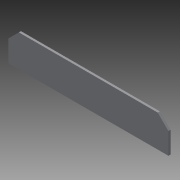
# Autodesk Inventor part: autorzy projektu
Saved by Autodesk Inventor 2014 (Build 180170000, 170)
## iProperties
Created: 2018-03-11
Part Number: autorzy projektu
Material: Generic
Document SubType Name: Modeling
Designer: HP820
Density: 1 g/cm^3
Appearance: Default
Author: HP820
Autodesk Inventor part; units mm, degrees
ref_plane "YZ Plane" through (0, 0, 0) normal (1, 0, 0) x (0, 1, 0)
ref_plane "XZ Plane" through (0, 0, 0) normal (0, 1, 0) x (-1, 0, 0)
ref_plane "XY Plane" through (0, 0, 0) normal (0, 0, 1) x (1, 0, 0)
sketch "Sketch1" plane through (0, 0, 0) normal (0, 1, 0) x (-1, 0, 0)
  line L0 (-75, 15) -> (75, 15)
  line L1 (75, 15) -> (75, -15)
  line L2 (75, -15) -> (-75, -15)
  line L3 (-75, -15) -> (-75, 15)
  line L4 (-75, 15) -> (75, -15) construction
  line L5 (75, 15) -> (-75, -15) construction
  point P0 (0, 0)
  dimension "d0" = 150
  dimension "d1" = 30
  constraints: 12 end point, 2 midpoint, 2 parallel, 1 horizontal, 1 perpendicular
  measures "d0" distance of L1.end L2.end
  measures "d1" distance of L0.end L1.end
extrude "Extrusion1" add sketch "Sketch1" along normal blind 2
chamfer "Chamfer1" distance 10 angle 45 2 edges at (75, 1, 15) (-75, 1, 15)
sketch "Sketch2" plane through (0, 2, 0) normal (0, 1, 0) x (1, 0, 0)
  line L0 (74.6856, -7.7413) -> (-73.3171, -7.7413) construction
  line L1 (-73.3171, -7.7413) -> (-73.3171, 7.0993) construction
  line L2 (-73.3171, 7.0993) -> (74.6856, 7.0993) construction
  line L3 (74.6856, 7.0993) -> (74.6856, -7.7413) construction
  spline S0 degree 2 poles (34.3952, -8.515) (34.3952, -8.0272) (35.3438, -8.0272) knots 0 0 0 1 1 1
  line L4 (35.3438, -8.0272) -> (37.8644, -8.0272)
  line L5 (37.8644, -8.0272) -> (37.8644, -6.1454)
  line L6 (37.8644, -6.1454) -> (39.4209, -6.1454)
  line L7 (39.4209, -6.1454) -> (39.4209, -11.3454)
  line L8 (39.4209, -11.3454) -> (35.3438, -11.3454)
  spline S1 degree 2 poles (35.3438, -11.3454) (34.3952, -11.3454) (34.3952, -10.8653) knots 0 0 0 1 1 1
  line L9 (34.3952, -10.8653) -> (34.3952, -8.515)
  line L10 (35.9633, -8.697) -> (35.9633, -10.6756)
  line L11 (35.9633, -10.6756) -> (37.8644, -10.6756)
  line L12 (37.8644, -10.6756) -> (37.8644, -8.697)
  line L13 (37.8644, -8.697) -> (35.9633, -8.697)
  line L14 (29.1371, -8.0969) -> (30.6433, -8.0969)
  line L15 (30.6433, -8.0969) -> (30.6433, -8.8674)
  line L16 (30.6433, -8.8674) -> (31.8474, -8.8519)
  line L17 (31.8474, -8.8519) -> (31.8474, -6.1454)
  line L18 (31.8474, -6.1454) -> (33.3691, -6.1454)
  line L19 (33.3691, -6.1454) -> (33.3691, -9.4985)
  line L20 (33.3691, -9.4985) -> (31.8474, -9.4985)
  line L21 (31.8474, -9.4985) -> (31.8474, -9.3785)
  spline S2 degree 2 poles (31.8474, -9.3785) (31.3751, -9.4211) (30.9104, -9.4637) knots 0 0 0 1 1 1
  spline S3 degree 2 poles (30.9104, -9.4637) (30.3451, -9.514) (29.9657, -9.514) knots 0 0 0 1 1 1
  spline S4 degree 2 poles (29.9657, -9.514) (29.1371, -9.514) (29.1371, -9.1036) knots 0 0 0 1 1 1
  line L22 (29.1371, -9.1036) -> (29.1371, -8.0969)
  spline S5 degree 2 poles (23.8519, -6.5597) (23.8519, -6.1454) (24.696, -6.1454) knots 0 0 0 1 1 1
  line L23 (24.696, -6.1454) -> (27.4218, -6.1454)
  spline S6 degree 2 poles (27.4218, -6.1454) (28.2775, -6.1454) (28.2775, -6.5597) knots 0 0 0 1 1 1
  line L24 (28.2775, -6.5597) -> (28.2775, -9.0842)
  spline S7 degree 2 poles (28.2775, -9.0842) (28.2775, -9.4985) (27.4218, -9.4985) knots 0 0 0 1 1 1
  line L25 (27.4218, -9.4985) -> (24.696, -9.4985)
  spline S8 degree 2 poles (24.696, -9.4985) (23.8519, -9.4985) (23.8519, -9.0842) knots 0 0 0 1 1 1
  line L26 (23.8519, -9.0842) -> (23.8519, -6.5597)
  line L27 (25.3387, -6.7765) -> (25.3387, -8.8674)
  line L28 (25.3387, -8.8674) -> (26.783, -8.8674)
  line L29 (26.783, -8.8674) -> (26.783, -6.7765)
  line L30 (26.783, -6.7765) -> (25.3387, -6.7765)
  spline S9 degree 2 poles (21.219, -5.3362) (21.219, -4.918) (22.0631, -4.918) knots 0 0 0 1 1 1
  line L31 (22.0631, -4.918) -> (23.6777, -4.918)
  line L32 (23.6777, -4.918) -> (23.6777, -5.553)
  line L33 (23.6777, -5.553) -> (22.7136, -5.553)
  line L34 (22.7136, -5.553) -> (22.7136, -9.4985)
  line L35 (22.7136, -9.4985) -> (21.219, -9.4985)
  line L36 (21.219, -9.4985) -> (21.219, -5.3362)
  line L37 (21.2035, -9.9825) -> (22.7252, -9.9825)
  line L38 (22.7252, -9.9825) -> (22.7252, -10.7646)
  line L39 (22.7252, -10.7646) -> (21.2035, -10.7646)
  line L40 (21.2035, -10.7646) -> (21.2035, -9.9825)
  spline S10 degree 2 poles (15.7441, -6.5597) (15.7441, -6.1454) (16.6037, -6.1454) knots 0 0 0 1 1 1
  line L41 (16.6037, -6.1454) -> (19.2288, -6.1454)
  spline S11 degree 2 poles (19.2288, -6.1454) (20.0845, -6.1454) (20.0845, -6.5597) knots 0 0 0 1 1 1
  line L42 (20.0845, -6.5597) -> (20.0845, -9.0842)
  spline S12 degree 2 poles (20.0845, -9.0842) (20.0845, -9.4985) (19.2288, -9.4985) knots 0 0 0 1 1 1
  line L43 (19.2288, -9.4985) -> (16.6037, -9.4985)
  spline S13 degree 2 poles (16.6037, -9.4985) (15.7441, -9.4985) (15.7441, -9.0842) knots 0 0 0 1 1 1
  line L44 (15.7441, -9.0842) -> (15.7441, -7.8529)
  line L45 (15.7441, -7.8529) -> (16.1623, -7.6438)
  line L46 (16.1623, -7.6438) -> (18.6287, -7.6438)
  line L47 (18.6287, -7.6438) -> (18.6287, -6.703)
  line L48 (18.6287, -6.703) -> (17.1999, -6.703)
  line L49 (17.1999, -6.703) -> (17.1999, -7.2605)
  line L50 (17.1999, -7.2605) -> (15.7441, -7.2605)
  line L51 (15.7441, -7.2605) -> (15.7441, -6.5597)
  line L52 (17.1999, -8.1395) -> (17.1999, -8.9409)
  line L53 (17.1999, -8.9409) -> (18.6287, -8.9409)
  line L54 (18.6287, -8.9409) -> (18.6287, -8.1395)
  line L55 (18.6287, -8.1395) -> (17.1999, -8.1395)
  line L56 (10.1608, -6.1454) -> (11.7831, -6.1454)
  line L57 (11.7831, -6.1454) -> (13.1189, -7.6826)
  line L58 (13.1189, -7.6826) -> (13.1189, -6.1454)
  line L59 (13.1189, -6.1454) -> (14.6406, -6.1454)
  line L60 (14.6406, -6.1454) -> (14.6406, -11.3454)
  line L61 (14.6406, -11.3454) -> (13.1189, -11.3454)
  line L62 (13.1189, -11.3454) -> (13.1189, -8.2208)
  line L63 (13.1189, -8.2208) -> (11.9148, -9.4985)
  line L64 (11.9148, -9.4985) -> (10.3273, -9.4985)
  line L65 (10.3273, -9.4985) -> (10.3273, -9.4869)
  line L66 (10.3273, -9.4869) -> (11.876, -7.9613)
  line L67 (11.876, -7.9613) -> (10.1608, -6.1454)
  line L68 (6.6102, -6.1454) -> (8.2984, -6.1454)
  spline S14 degree 2 poles (8.2984, -6.1454) (9.1425, -6.1454) (9.1425, -6.5597) knots 0 0 0 1 1 1
  line L69 (9.1425, -6.5597) -> (9.1425, -8.8519)
  line L70 (9.1425, -8.8519) -> (9.8588, -8.8519)
  line L71 (9.8588, -8.8519) -> (9.8588, -9.4985)
  line L72 (9.8588, -9.4985) -> (9.1425, -9.4985)
  line L73 (9.1425, -9.4985) -> (9.1425, -10.4123)
  line L74 (9.1425, -10.4123) -> (7.6247, -10.4123)
  line L75 (7.6247, -10.4123) -> (7.6247, -9.4985)
  line L76 (7.6247, -9.4985) -> (6.6489, -9.4985)
  line L77 (6.6489, -9.4985) -> (6.6489, -8.8519)
  line L78 (6.6489, -8.8519) -> (7.6247, -8.8519)
  line L79 (7.6247, -8.8519) -> (7.6247, -6.792)
  line L80 (7.6247, -6.792) -> (6.6102, -6.792)
  line L81 (6.6102, -6.792) -> (6.6102, -6.1454)
  line L82 (-3.6852, -9.4985) -> (-2.241, -6.1377)
  line L83 (-2.241, -6.1377) -> (-0.9129, -6.1377)
  line L84 (-0.9129, -6.1377) -> (-0.1889, -7.9962)
  line L85 (-0.1889, -7.9962) -> (0.5352, -6.1377)
  line L86 (0.5352, -6.1377) -> (1.8516, -6.1377)
  line L87 (1.8516, -6.1377) -> (3.2958, -9.4985)
  line L88 (3.2958, -9.4985) -> (1.84, -9.4985)
  line L89 (1.84, -9.4985) -> (1.1082, -7.3573)
  line L90 (1.1082, -7.3573) -> (0.3842, -9.4985)
  line L91 (0.3842, -9.4985) -> (-0.7736, -9.4985)
  line L92 (-0.7736, -9.4985) -> (-1.4976, -7.3573)
  line L93 (-1.4976, -7.3573) -> (-2.2294, -9.4985)
  line L94 (-2.2294, -9.4985) -> (-3.6852, -9.4985)
  line L95 (-8.982, -9.4985) -> (-7.3016, -6.188)
  line L96 (-7.3016, -6.188) -> (-6.655, -4.918)
  line L97 (-6.655, -4.918) -> (-5.0985, -4.918)
  line L98 (-5.0985, -4.918) -> (-5.7993, -6.1725)
  line L99 (-5.7993, -6.1725) -> (-4.0957, -9.4985)
  line L100 (-4.0957, -9.4985) -> (-5.6599, -9.4985)
  line L101 (-5.6599, -9.4985) -> (-6.5427, -7.2954)
  line L102 (-6.5427, -7.2954) -> (-7.4255, -9.4985)
  line L103 (-7.4255, -9.4985) -> (-8.982, -9.4985)
  line L104 (-14.213, -6.1454) -> (-12.5907, -6.1454)
  line L105 (-12.5907, -6.1454) -> (-11.2549, -7.6826)
  line L106 (-11.2549, -7.6826) -> (-11.2549, -6.1454)
  line L107 (-11.2549, -6.1454) -> (-9.7332, -6.1454)
  line L108 (-9.7332, -6.1454) -> (-9.7332, -11.3454)
  line L109 (-9.7332, -11.3454) -> (-11.2549, -11.3454)
  line L110 (-11.2549, -11.3454) -> (-11.2549, -8.2208)
  line L111 (-11.2549, -8.2208) -> (-12.459, -9.4985)
  line L112 (-12.459, -9.4985) -> (-14.0465, -9.4985)
  line L113 (-14.0465, -9.4985) -> (-14.0465, -9.4869)
  line L114 (-14.0465, -9.4869) -> (-12.4978, -7.9613)
  line L115 (-12.4978, -7.9613) -> (-14.213, -6.1454)
  spline S15 degree 2 poles (-19.293, -6.5597) (-19.293, -6.1454) (-18.4489, -6.1454) knots 0 0 0 1 1 1
  line L116 (-18.4489, -6.1454) -> (-15.7231, -6.1454)
  spline S16 degree 2 poles (-15.7231, -6.1454) (-14.8674, -6.1454) (-14.8674, -6.5597) knots 0 0 0 1 1 1
  line L117 (-14.8674, -6.5597) -> (-14.8674, -9.0842)
  spline S17 degree 2 poles (-14.8674, -9.0842) (-14.8674, -9.4985) (-15.7231, -9.4985) knots 0 0 0 1 1 1
  line L118 (-15.7231, -9.4985) -> (-18.4489, -9.4985)
  spline S18 degree 2 poles (-18.4489, -9.4985) (-19.293, -9.4985) (-19.293, -9.0842) knots 0 0 0 1 1 1
  line L119 (-19.293, -9.0842) -> (-19.293, -6.5597)
  line L120 (-17.8062, -6.7765) -> (-17.8062, -8.8674)
  line L121 (-17.8062, -8.8674) -> (-16.3619, -8.8674)
  line L122 (-16.3619, -8.8674) -> (-16.3619, -6.7765)
  line L123 (-16.3619, -6.7765) -> (-17.8062, -6.7765)
  line L124 (-24.8724, -6.1454) -> (-23.343, -6.1454)
  line L125 (-23.343, -6.1454) -> (-23.343, -8.8674)
  line L126 (-23.343, -8.8674) -> (-21.9143, -8.8519)
  line L127 (-21.9143, -8.8519) -> (-21.9143, -6.1454)
  line L128 (-21.9143, -6.1454) -> (-20.3926, -6.1454)
  line L129 (-20.3926, -6.1454) -> (-20.3926, -9.4985)
  line L130 (-20.3926, -9.4985) -> (-21.9143, -9.4985)
  line L131 (-21.9143, -9.4985) -> (-21.9143, -9.3785)
  spline S19 degree 2 poles (-21.9143, -9.3785) (-22.4447, -9.4211) (-22.9713, -9.4598) knots 0 0 0 1 1 1
  spline S20 degree 2 poles (-22.9713, -9.4598) (-23.6218, -9.514) (-24.04, -9.514) knots 0 0 0 1 1 1
  spline S21 degree 2 poles (-24.04, -9.514) (-24.8724, -9.514) (-24.8724, -9.1036) knots 0 0 0 1 1 1
  line L132 (-24.8724, -9.1036) -> (-24.8724, -6.1454)
  line L133 (-30.2893, -6.1454) -> (-28.8334, -6.1454)
  line L134 (-28.8334, -6.1454) -> (-28.8334, -6.2616)
  spline S22 degree 2 poles (-28.8334, -6.2616) (-28.3185, -6.2228) (-27.7996, -6.1803) knots 0 0 0 1 1 1
  spline S23 degree 2 poles (-27.7996, -6.1803) (-27.122, -6.1338) (-26.7697, -6.1338) knots 0 0 0 1 1 1
  spline S24 degree 2 poles (-26.7697, -6.1338) (-25.9372, -6.1338) (-25.9372, -6.5403) knots 0 0 0 1 1 1
  line L135 (-25.9372, -6.5403) -> (-25.9372, -7.7484)
  spline S25 degree 2 poles (-25.9372, -7.7484) (-25.9372, -8.1666) (-26.7929, -8.1666) knots 0 0 0 1 1 1
  line L136 (-26.7929, -8.1666) -> (-28.8489, -8.1666)
  line L137 (-28.8489, -8.1666) -> (-28.8489, -8.9371)
  line L138 (-28.8489, -8.9371) -> (-27.3931, -8.9371)
  line L139 (-27.3931, -8.9371) -> (-27.3931, -8.457)
  line L140 (-27.3931, -8.457) -> (-26.0185, -8.457)
  line L141 (-26.0185, -8.457) -> (-26.0185, -9.0842)
  spline S26 degree 2 poles (-26.0185, -9.0842) (-26.0185, -9.4985) (-26.8742, -9.4985) knots 0 0 0 1 1 1
  line L142 (-26.8742, -9.4985) -> (-29.4452, -9.4985)
  spline S27 degree 2 poles (-29.4452, -9.4985) (-30.2893, -9.4985) (-30.2893, -9.0842) knots 0 0 0 1 1 1
  line L143 (-30.2893, -9.0842) -> (-30.2893, -6.1454)
  line L144 (-28.8489, -6.7494) -> (-28.8489, -7.6516)
  line L145 (-28.8489, -7.6516) -> (-27.3931, -7.6516)
  line L146 (-27.3931, -7.6516) -> (-27.3931, -6.7223)
  line L147 (-27.3931, -6.7223) -> (-28.8489, -6.7494)
  line L148 (-32.9144, -6.1454) -> (-31.4199, -6.1454)
  line L149 (-31.4199, -6.1454) -> (-31.4199, -11.3454)
  line L150 (-31.4199, -11.3454) -> (-32.9144, -11.3454)
  line L151 (-32.9144, -11.3454) -> (-32.9144, -6.1454)
  line L152 (-35.5822, -6.1454) -> (-34.0876, -6.1454)
  line L153 (-34.0876, -6.1454) -> (-34.0876, -9.4985)
  line L154 (-34.0876, -9.4985) -> (-35.5822, -9.4985)
  line L155 (-35.5822, -9.4985) -> (-35.5822, -6.1454)
  line L156 (-35.5977, -9.9825) -> (-34.076, -9.9825)
  line L157 (-34.076, -9.9825) -> (-34.076, -10.7646)
  line L158 (-34.076, -10.7646) -> (-35.5977, -10.7646)
  line L159 (-35.5977, -10.7646) -> (-35.5977, -9.9825)
  line L160 (-38.1725, -8.2556) -> (-36.6741, -8.2556)
  line L161 (-36.6741, -8.2556) -> (-36.6741, -9.0648)
  line L162 (-36.6741, -9.0648) -> (-38.1725, -9.0648)
  line L163 (-38.1725, -9.0648) -> (-38.1725, -8.2556)
  line L164 (-38.1725, -6.1454) -> (-36.6741, -6.1454)
  line L165 (-36.6741, -6.1454) -> (-36.6741, -6.9508)
  line L166 (-36.6741, -6.9508) -> (-38.1725, -6.9508)
  line L167 (-38.1725, -6.9508) -> (-38.1725, -6.1454)
  spline S28 degree 2 poles (33.3943, 1.7931) (33.3943, 2.2693) (34.3506, 2.2693) knots 0 0 0 1 1 1
  line L168 (34.3506, 2.2693) -> (37.3011, 2.2693)
  spline S29 degree 2 poles (37.3011, 2.2693) (38.2381, 2.2693) (38.2381, 1.7931) knots 0 0 0 1 1 1
  line L169 (38.2381, 1.7931) -> (38.2381, 0.5154)
  line L170 (38.2381, 0.5154) -> (36.6893, 0.5154)
  line L171 (36.6893, 0.5154) -> (36.6893, 1.6034)
  line L172 (36.6893, 1.6034) -> (34.9469, 1.6034)
  line L173 (34.9469, 1.6034) -> (34.9469, -2.9307)
  line L174 (34.9469, -2.9307) -> (33.3943, -2.9307)
  line L175 (33.3943, -2.9307) -> (33.3943, 1.7931)
  line L176 (27.9116, 2.2693) -> (29.3675, 2.2693)
  line L177 (29.3675, 2.2693) -> (29.3675, 2.1532)
  spline S30 degree 2 poles (29.3675, 2.1532) (29.8824, 2.1919) (30.4013, 2.2345) knots 0 0 0 1 1 1
  spline S31 degree 2 poles (30.4013, 2.2345) (31.0789, 2.281) (31.4312, 2.281) knots 0 0 0 1 1 1
  spline S32 degree 2 poles (31.4312, 2.281) (32.2637, 2.281) (32.2637, 1.8744) knots 0 0 0 1 1 1
  line L178 (32.2637, 1.8744) -> (32.2637, 0.6664)
  spline S33 degree 2 poles (32.2637, 0.6664) (32.2637, 0.2482) (31.408, 0.2482) knots 0 0 0 1 1 1
  line L179 (31.408, 0.2482) -> (29.352, 0.2482)
  line L180 (29.352, 0.2482) -> (29.352, -0.5223)
  line L181 (29.352, -0.5223) -> (30.8078, -0.5223)
  line L182 (30.8078, -0.5223) -> (30.8078, -0.0422)
  line L183 (30.8078, -0.0422) -> (32.1824, -0.0422)
  line L184 (32.1824, -0.0422) -> (32.1824, -0.6695)
  spline S34 degree 2 poles (32.1824, -0.6695) (32.1824, -1.0838) (31.3267, -1.0838) knots 0 0 0 1 1 1
  line L185 (31.3267, -1.0838) -> (28.7557, -1.0838)
  spline S35 degree 2 poles (28.7557, -1.0838) (27.9116, -1.0838) (27.9116, -0.6695) knots 0 0 0 1 1 1
  line L186 (27.9116, -0.6695) -> (27.9116, 2.2693)
  line L187 (29.352, 1.6653) -> (29.352, 0.7632)
  line L188 (29.352, 0.7632) -> (30.8078, 0.7632)
  line L189 (30.8078, 0.7632) -> (30.8078, 1.6924)
  line L190 (30.8078, 1.6924) -> (29.352, 1.6653)
  spline S36 degree 2 poles (22.4793, 1.855) (22.4793, 2.2693) (23.3234, 2.2693) knots 0 0 0 1 1 1
  line L191 (23.3234, 2.2693) -> (25.964, 2.2693)
  spline S37 degree 2 poles (25.964, 2.2693) (26.8197, 2.2693) (26.8197, 1.855) knots 0 0 0 1 1 1
  line L192 (26.8197, 1.855) -> (26.8197, -0.6695)
  spline S38 degree 2 poles (26.8197, -0.6695) (26.8197, -1.0838) (25.964, -1.0838) knots 0 0 0 1 1 1
  line L193 (25.964, -1.0838) -> (23.3234, -1.0838)
  spline S39 degree 2 poles (23.3234, -1.0838) (22.4793, -1.0838) (22.4793, -0.6695) knots 0 0 0 1 1 1
  line L194 (22.4793, -0.6695) -> (22.4793, 0.1282)
  line L195 (22.4793, 0.1282) -> (23.9623, 0.1282)
  line L196 (23.9623, 0.1282) -> (23.9623, -0.4526)
  line L197 (23.9623, -0.4526) -> (25.3252, -0.4526)
  line L198 (25.3252, -0.4526) -> (25.3252, 1.6382)
  line L199 (25.3252, 1.6382) -> (23.9623, 1.6382)
  line L200 (23.9623, 1.6382) -> (23.9623, 0.9955)
  line L201 (23.9623, 0.9955) -> (22.4793, 0.9955)
  line L202 (22.4793, 0.9955) -> (22.4793, 1.855)
  spline S40 degree 2 poles (17.047, 1.855) (17.047, 2.2693) (17.9066, 2.2693) knots 0 0 0 1 1 1
  line L203 (17.9066, 2.2693) -> (20.5317, 2.2693)
  spline S41 degree 2 poles (20.5317, 2.2693) (21.3874, 2.2693) (21.3874, 1.855) knots 0 0 0 1 1 1
  line L204 (21.3874, 1.855) -> (21.3874, -0.6695)
  spline S42 degree 2 poles (21.3874, -0.6695) (21.3874, -1.0838) (20.5317, -1.0838) knots 0 0 0 1 1 1
  line L205 (20.5317, -1.0838) -> (17.9066, -1.0838)
  spline S43 degree 2 poles (17.9066, -1.0838) (17.047, -1.0838) (17.047, -0.6695) knots 0 0 0 1 1 1
  line L206 (17.047, -0.6695) -> (17.047, 0.5618)
  line L207 (17.047, 0.5618) -> (17.4652, 0.7709)
  line L208 (17.4652, 0.7709) -> (19.9316, 0.7709)
  line L209 (19.9316, 0.7709) -> (19.9316, 1.7118)
  line L210 (19.9316, 1.7118) -> (18.5028, 1.7118)
  line L211 (18.5028, 1.7118) -> (18.5028, 1.1542)
  line L212 (18.5028, 1.1542) -> (17.047, 1.1542)
  line L213 (17.047, 1.1542) -> (17.047, 1.855)
  line L214 (18.5028, 0.2753) -> (18.5028, -0.5262)
  line L215 (18.5028, -0.5262) -> (19.9316, -0.5262)
  line L216 (19.9316, -0.5262) -> (19.9316, 0.2753)
  line L217 (19.9316, 0.2753) -> (18.5028, 0.2753)
  line L218 (11.4637, 2.2693) -> (13.086, 2.2693)
  line L219 (13.086, 2.2693) -> (14.4218, 0.7322)
  line L220 (14.4218, 0.7322) -> (14.4218, 2.2693)
  line L221 (14.4218, 2.2693) -> (15.9435, 2.2693)
  line L222 (15.9435, 2.2693) -> (15.9435, -2.9307)
  line L223 (15.9435, -2.9307) -> (14.4218, -2.9307)
  line L224 (14.4218, -2.9307) -> (14.4218, 0.194)
  line L225 (14.4218, 0.194) -> (13.2177, -1.0838)
  line L226 (13.2177, -1.0838) -> (11.6302, -1.0838)
  line L227 (11.6302, -1.0838) -> (11.6302, -1.0721)
  line L228 (11.6302, -1.0721) -> (13.1789, 0.4534)
  line L229 (13.1789, 0.4534) -> (11.4637, 2.2693)
  line L230 (1.6367, 2.2693) -> (3.1313, 2.2693)
  line L231 (3.1313, 2.2693) -> (3.1313, -0.2939)
  spline S44 degree 2 poles (3.1313, -0.2939) (3.1313, -0.4991) (3.0384, -0.8592) knots 0 0 0 1 1 1
  line L232 (3.0384, -0.8592) -> (4.3819, 1.7931)
  line L233 (4.3819, 1.7931) -> (5.1718, 1.7931)
  line L234 (5.1718, 1.7931) -> (6.5192, -0.8592)
  spline S45 degree 2 poles (6.5192, -0.8592) (6.4263, -0.4913) (6.4263, -0.2939) knots 0 0 0 1 1 1
  line L235 (6.4263, -0.2939) -> (6.4263, 2.2693)
  line L236 (6.4263, 2.2693) -> (7.9247, 2.2693)
  line L237 (7.9247, 2.2693) -> (7.9247, -2.9307)
  line L238 (7.9247, -2.9307) -> (6.4534, -2.9307)
  line L239 (6.4534, -2.9307) -> (4.8194, -0.0577)
  spline S46 degree 2 poles (4.8194, -0.0577) (4.7923, -0.0112) (4.7807, 0.1785) knots 0 0 0 1 1 1
  spline S47 degree 2 poles (4.7807, 0.1785) (4.7807, 0.0972) (4.7381, -0.0577) knots 0 0 0 1 1 1
  line L240 (4.7381, -0.0577) -> (3.1042, -2.9307)
  line L241 (3.1042, -2.9307) -> (1.6367, -2.9307)
  line L242 (1.6367, -2.9307) -> (1.6367, 2.2693)
  line L243 (-3.8537, 2.2693) -> (-2.3978, 2.2693)
  line L244 (-2.3978, 2.2693) -> (-2.3978, 2.1532)
  spline S48 degree 2 poles (-2.3978, 2.1532) (-1.8829, 2.1919) (-1.364, 2.2345) knots 0 0 0 1 1 1
  spline S49 degree 2 poles (-1.364, 2.2345) (-0.6864, 2.281) (-0.3341, 2.281) knots 0 0 0 1 1 1
  spline S50 degree 2 poles (-0.3341, 2.281) (0.4984, 2.281) (0.4984, 1.8744) knots 0 0 0 1 1 1
  line L245 (0.4984, 1.8744) -> (0.4984, 0.6664)
  spline S51 degree 2 poles (0.4984, 0.6664) (0.4984, 0.2482) (-0.3573, 0.2482) knots 0 0 0 1 1 1
  line L246 (-0.3573, 0.2482) -> (-2.4133, 0.2482)
  line L247 (-2.4133, 0.2482) -> (-2.4133, -0.5223)
  line L248 (-2.4133, -0.5223) -> (-0.9575, -0.5223)
  line L249 (-0.9575, -0.5223) -> (-0.9575, -0.0422)
  line L250 (-0.9575, -0.0422) -> (0.4171, -0.0422)
  line L251 (0.4171, -0.0422) -> (0.4171, -0.6695)
  spline S52 degree 2 poles (0.4171, -0.6695) (0.4171, -1.0838) (-0.4386, -1.0838) knots 0 0 0 1 1 1
  line L252 (-0.4386, -1.0838) -> (-3.0096, -1.0838)
  spline S53 degree 2 poles (-3.0096, -1.0838) (-3.8537, -1.0838) (-3.8537, -0.6695) knots 0 0 0 1 1 1
  line L253 (-3.8537, -0.6695) -> (-3.8537, 2.2693)
  line L254 (-2.4133, 1.6653) -> (-2.4133, 0.7632)
  line L255 (-2.4133, 0.7632) -> (-0.9575, 0.7632)
  line L256 (-0.9575, 0.7632) -> (-0.9575, 1.6924)
  line L257 (-0.9575, 1.6924) -> (-2.4133, 1.6653)
  line L258 (-9.1776, 0.3179) -> (-7.6714, 0.3179)
  line L259 (-7.6714, 0.3179) -> (-7.6714, -0.4526)
  line L260 (-7.6714, -0.4526) -> (-6.4672, -0.4371)
  line L261 (-6.4672, -0.4371) -> (-6.4672, 2.2693)
  line L262 (-6.4672, 2.2693) -> (-4.9456, 2.2693)
  line L263 (-4.9456, 2.2693) -> (-4.9456, -1.0838)
  line L264 (-4.9456, -1.0838) -> (-6.4672, -1.0838)
  line L265 (-6.4672, -1.0838) -> (-6.4672, -0.9637)
  spline S54 degree 2 poles (-6.4672, -0.9637) (-6.9396, -1.0063) (-7.4042, -1.0489) knots 0 0 0 1 1 1
  spline S55 degree 2 poles (-7.4042, -1.0489) (-7.9695, -1.0992) (-8.349, -1.0992) knots 0 0 0 1 1 1
  spline S56 degree 2 poles (-8.349, -1.0992) (-9.1776, -1.0992) (-9.1776, -0.6888) knots 0 0 0 1 1 1
  line L266 (-9.1776, -0.6888) -> (-9.1776, 0.3179)
  line L267 (-12.9333, 2.2693) -> (-11.2452, 2.2693)
  spline S57 degree 2 poles (-11.2452, 2.2693) (-10.4011, 2.2693) (-10.4011, 1.855) knots 0 0 0 1 1 1
  line L268 (-10.4011, 1.855) -> (-10.4011, -0.4371)
  line L269 (-10.4011, -0.4371) -> (-9.6848, -0.4371)
  line L270 (-9.6848, -0.4371) -> (-9.6848, -1.0838)
  line L271 (-9.6848, -1.0838) -> (-10.4011, -1.0838)
  line L272 (-10.4011, -1.0838) -> (-10.4011, -1.9975)
  line L273 (-10.4011, -1.9975) -> (-11.9189, -1.9975)
  line L274 (-11.9189, -1.9975) -> (-11.9189, -1.0838)
  line L275 (-11.9189, -1.0838) -> (-12.8946, -1.0838)
  line L276 (-12.8946, -1.0838) -> (-12.8946, -0.4371)
  line L277 (-12.8946, -0.4371) -> (-11.9189, -0.4371)
  line L278 (-11.9189, -0.4371) -> (-11.9189, 1.6227)
  line L279 (-11.9189, 1.6227) -> (-12.9333, 1.6227)
  line L280 (-12.9333, 1.6227) -> (-12.9333, 2.2693)
  line L281 (-18.3269, -1.0838) -> (-16.6465, 2.2267)
  line L282 (-16.6465, 2.2267) -> (-15.9999, 3.4967)
  line L283 (-15.9999, 3.4967) -> (-14.4434, 3.4967)
  line L284 (-14.4434, 3.4967) -> (-15.1442, 2.2422)
  line L285 (-15.1442, 2.2422) -> (-13.4406, -1.0838)
  line L286 (-13.4406, -1.0838) -> (-15.0048, -1.0838)
  line L287 (-15.0048, -1.0838) -> (-15.8876, 1.1194)
  line L288 (-15.8876, 1.1194) -> (-16.7704, -1.0838)
  line L289 (-16.7704, -1.0838) -> (-18.3269, -1.0838)
  line L290 (-23.5579, 2.2693) -> (-22.0285, 2.2693)
  line L291 (-22.0285, 2.2693) -> (-22.0285, -0.4526)
  line L292 (-22.0285, -0.4526) -> (-20.5998, -0.4371)
  line L293 (-20.5998, -0.4371) -> (-20.5998, 2.2693)
  line L294 (-20.5998, 2.2693) -> (-19.0781, 2.2693)
  line L295 (-19.0781, 2.2693) -> (-19.0781, -1.0838)
  line L296 (-19.0781, -1.0838) -> (-20.5998, -1.0838)
  line L297 (-20.5998, -1.0838) -> (-20.5998, -0.9637)
  spline S58 degree 2 poles (-20.5998, -0.9637) (-21.1302, -1.0063) (-21.6568, -1.045) knots 0 0 0 1 1 1
  spline S59 degree 2 poles (-21.6568, -1.045) (-22.3073, -1.0992) (-22.7255, -1.0992) knots 0 0 0 1 1 1
  spline S60 degree 2 poles (-22.7255, -1.0992) (-23.5579, -1.0992) (-23.5579, -0.6888) knots 0 0 0 1 1 1
  line L298 (-23.5579, -0.6888) -> (-23.5579, 2.2693)
  line L299 (-26.1831, 2.2693) -> (-24.6885, 2.2693)
  line L300 (-24.6885, 2.2693) -> (-24.6885, -1.0838)
  line L301 (-24.6885, -1.0838) -> (-26.1831, -1.0838)
  line L302 (-26.1831, -1.0838) -> (-26.1831, 2.2693)
  line L303 (-26.1986, -1.5677) -> (-24.6769, -1.5677)
  line L304 (-24.6769, -1.5677) -> (-24.6769, -2.3499)
  line L305 (-24.6769, -2.3499) -> (-26.1986, -2.3499)
  line L306 (-26.1986, -2.3499) -> (-26.1986, -1.5677)
  line L307 (-31.6425, 2.2693) -> (-30.1867, 2.2693)
  line L308 (-30.1867, 2.2693) -> (-30.1867, 2.1532)
  spline S61 degree 2 poles (-30.1867, 2.1532) (-29.6717, 2.1919) (-29.1529, 2.2345) knots 0 0 0 1 1 1
  spline S62 degree 2 poles (-29.1529, 2.2345) (-28.4753, 2.281) (-28.1229, 2.281) knots 0 0 0 1 1 1
  spline S63 degree 2 poles (-28.1229, 2.281) (-27.2905, 2.281) (-27.2905, 1.8744) knots 0 0 0 1 1 1
  line L309 (-27.2905, 1.8744) -> (-27.2905, 0.6664)
  spline S64 degree 2 poles (-27.2905, 0.6664) (-27.2905, 0.2482) (-28.1462, 0.2482) knots 0 0 0 1 1 1
  line L310 (-28.1462, 0.2482) -> (-30.2021, 0.2482)
  line L311 (-30.2021, 0.2482) -> (-30.2021, -0.5223)
  line L312 (-30.2021, -0.5223) -> (-28.7463, -0.5223)
  line L313 (-28.7463, -0.5223) -> (-28.7463, -0.0422)
  line L314 (-28.7463, -0.0422) -> (-27.3718, -0.0422)
  line L315 (-27.3718, -0.0422) -> (-27.3718, -0.6695)
  spline S65 degree 2 poles (-27.3718, -0.6695) (-27.3718, -1.0838) (-28.2275, -1.0838) knots 0 0 0 1 1 1
  line L316 (-28.2275, -1.0838) -> (-30.7984, -1.0838)
  spline S66 degree 2 poles (-30.7984, -1.0838) (-31.6425, -1.0838) (-31.6425, -0.6695) knots 0 0 0 1 1 1
  line L317 (-31.6425, -0.6695) -> (-31.6425, 2.2693)
  line L318 (-30.2021, 1.6653) -> (-30.2021, 0.7632)
  line L319 (-30.2021, 0.7632) -> (-28.7463, 0.7632)
  line L320 (-28.7463, 0.7632) -> (-28.7463, 1.6924)
  line L321 (-28.7463, 1.6924) -> (-30.2021, 1.6653)
  line L322 (-37.2142, 2.2693) -> (-35.5919, 2.2693)
  line L323 (-35.5919, 2.2693) -> (-34.2561, 0.7322)
  line L324 (-34.2561, 0.7322) -> (-34.2561, 2.2693)
  line L325 (-34.2561, 2.2693) -> (-32.7344, 2.2693)
  line L326 (-32.7344, 2.2693) -> (-32.7344, -2.9307)
  line L327 (-32.7344, -2.9307) -> (-34.2561, -2.9307)
  line L328 (-34.2561, -2.9307) -> (-34.2561, 0.194)
  line L329 (-34.2561, 0.194) -> (-35.4602, -1.0838)
  line L330 (-35.4602, -1.0838) -> (-37.0477, -1.0838)
  line L331 (-37.0477, -1.0838) -> (-37.0477, -1.0721)
  line L332 (-37.0477, -1.0721) -> (-35.4989, 0.4534)
  line L333 (-35.4989, 0.4534) -> (-37.2142, 2.2693)
  line L334 (44.6558, 10.6841) -> (48.7445, 10.6841)
  line L335 (48.7445, 10.6841) -> (48.7445, 5.4841)
  line L336 (48.7445, 5.4841) -> (47.188, 5.4841)
  line L337 (47.188, 5.4841) -> (47.188, 9.991)
  line L338 (47.188, 9.991) -> (44.6558, 9.991)
  line L339 (44.6558, 9.991) -> (44.6558, 10.6841)
  line L340 (45.7864, 7.9544) -> (49.3292, 9.0308)
  line L341 (49.3292, 9.0308) -> (49.3292, 8.4035)
  line L342 (49.3292, 8.4035) -> (45.7864, 7.331)
  line L343 (45.7864, 7.331) -> (45.7864, 7.9544)
  line L344 (39.3435, 10.6841) -> (40.8574, 10.6841)
  line L345 (40.8574, 10.6841) -> (40.8574, 10.5679)
  spline S67 degree 2 poles (40.8574, 10.5679) (41.384, 10.6105) (41.9145, 10.6531) knots 0 0 0 1 1 1
  spline S68 degree 2 poles (41.9145, 10.6531) (42.5572, 10.7034) (42.9792, 10.7034) knots 0 0 0 1 1 1
  spline S69 degree 2 poles (42.9792, 10.7034) (43.8078, 10.7034) (43.8078, 10.2891) knots 0 0 0 1 1 1
  line L346 (43.8078, 10.2891) -> (43.8078, 7.331)
  line L347 (43.8078, 7.331) -> (42.3016, 7.331)
  line L348 (42.3016, 7.331) -> (42.3016, 10.053)
  line L349 (42.3016, 10.053) -> (40.8574, 10.0375)
  line L350 (40.8574, 10.0375) -> (40.8574, 7.331)
  line L351 (40.8574, 7.331) -> (39.3435, 7.331)
  line L352 (39.3435, 7.331) -> (39.3435, 10.6841)
  line L353 (33.7563, 10.6841) -> (35.3786, 10.6841)
  line L354 (35.3786, 10.6841) -> (36.7145, 9.1469)
  line L355 (36.7145, 9.1469) -> (36.7145, 10.6841)
  line L356 (36.7145, 10.6841) -> (38.2361, 10.6841)
  line L357 (38.2361, 10.6841) -> (38.2361, 5.4841)
  line L358 (38.2361, 5.4841) -> (36.7145, 5.4841)
  line L359 (36.7145, 5.4841) -> (36.7145, 8.6087)
  line L360 (36.7145, 8.6087) -> (35.5103, 7.331)
  line L361 (35.5103, 7.331) -> (33.9228, 7.331)
  line L362 (33.9228, 7.331) -> (33.9228, 7.3426)
  line L363 (33.9228, 7.3426) -> (35.4716, 8.8682)
  line L364 (35.4716, 8.8682) -> (33.7563, 10.6841)
  line L365 (28.777, 10.6841) -> (30.2328, 10.6841)
  line L366 (30.2328, 10.6841) -> (30.2328, 10.5679)
  spline S70 degree 2 poles (30.2328, 10.5679) (30.7478, 10.6066) (31.2667, 10.6492) knots 0 0 0 1 1 1
  spline S71 degree 2 poles (31.2667, 10.6492) (31.9442, 10.6957) (32.2966, 10.6957) knots 0 0 0 1 1 1
  spline S72 degree 2 poles (32.2966, 10.6957) (33.129, 10.6957) (33.129, 10.2891) knots 0 0 0 1 1 1
  line L367 (33.129, 10.2891) -> (33.129, 9.0811)
  spline S73 degree 2 poles (33.129, 9.0811) (33.129, 8.6629) (32.2734, 8.6629) knots 0 0 0 1 1 1
  line L368 (32.2734, 8.6629) -> (30.2174, 8.6629)
  line L369 (30.2174, 8.6629) -> (30.2174, 7.8924)
  line L370 (30.2174, 7.8924) -> (31.6732, 7.8924)
  line L371 (31.6732, 7.8924) -> (31.6732, 8.3725)
  line L372 (31.6732, 8.3725) -> (33.0477, 8.3725)
  line L373 (33.0477, 8.3725) -> (33.0477, 7.7453)
  spline S74 degree 2 poles (33.0477, 7.7453) (33.0477, 7.331) (32.192, 7.331) knots 0 0 0 1 1 1
  line L374 (32.192, 7.331) -> (29.6211, 7.331)
  spline S75 degree 2 poles (29.6211, 7.331) (28.777, 7.331) (28.777, 7.7453) knots 0 0 0 1 1 1
  line L375 (28.777, 7.7453) -> (28.777, 10.6841)
  line L376 (30.2174, 10.0801) -> (30.2174, 9.1779)
  line L377 (30.2174, 9.1779) -> (31.6732, 9.1779)
  line L378 (31.6732, 9.1779) -> (31.6732, 10.1072)
  line L379 (31.6732, 10.1072) -> (30.2174, 10.0801)
  spline S76 degree 2 poles (23.4647, 10.2698) (23.4647, 10.6841) (24.3088, 10.6841) knots 0 0 0 1 1 1
  line L380 (24.3088, 10.6841) -> (26.8681, 10.6841)
  spline S77 degree 2 poles (26.8681, 10.6841) (27.7122, 10.6841) (27.7122, 10.2698) knots 0 0 0 1 1 1
  line L381 (27.7122, 10.2698) -> (27.7122, 9.5496)
  line L382 (27.7122, 9.5496) -> (26.2564, 9.5496)
  line L383 (26.2564, 9.5496) -> (26.2564, 10.111)
  line L384 (26.2564, 10.111) -> (24.9206, 10.111)
  line L385 (24.9206, 10.111) -> (24.9206, 9.5806)
  line L386 (24.9206, 9.5806) -> (27.2553, 8.8953)
  spline S78 degree 2 poles (27.2553, 8.8953) (27.7122, 8.7559) (27.7122, 8.5274) knots 0 0 0 1 1 1
  line L387 (27.7122, 8.5274) -> (27.7122, 7.7453)
  spline S79 degree 2 poles (27.7122, 7.7453) (27.7122, 7.331) (26.8565, 7.331) knots 0 0 0 1 1 1
  line L388 (26.8565, 7.331) -> (24.3243, 7.331)
  spline S80 degree 2 poles (24.3243, 7.331) (23.4763, 7.331) (23.4763, 7.7453) knots 0 0 0 1 1 1
  line L389 (23.4763, 7.7453) -> (23.4763, 8.419)
  line L390 (23.4763, 8.419) -> (24.9206, 8.419)
  line L391 (24.9206, 8.419) -> (24.9206, 7.9002)
  line L392 (24.9206, 7.9002) -> (26.2564, 7.9002)
  line L393 (26.2564, 7.9002) -> (26.2564, 8.3842)
  line L394 (26.2564, 8.3842) -> (23.9293, 9.0656)
  spline S81 degree 2 poles (23.9293, 9.0656) (23.4647, 9.2011) (23.4647, 9.4373) knots 0 0 0 1 1 1
  line L395 (23.4647, 9.4373) -> (23.4647, 10.2698)
  line L396 (18.6054, 10.6841) -> (22.6477, 10.6841)
  line L397 (22.6477, 10.6841) -> (22.6477, 10.2349)
  line L398 (22.6477, 10.2349) -> (20.4136, 7.9505)
  line L399 (20.4136, 7.9505) -> (22.4658, 7.9505)
  line L400 (22.4658, 7.9505) -> (22.4658, 7.331)
  line L401 (22.4658, 7.331) -> (18.6054, 7.331)
  line L402 (18.6054, 7.331) -> (18.6054, 7.7801)
  line L403 (18.6054, 7.7801) -> (20.8512, 10.0646)
  line L404 (20.8512, 10.0646) -> (18.6054, 10.0646)
  line L405 (18.6054, 10.0646) -> (18.6054, 10.6841)
  line L406 (9.5142, 10.6841) -> (10.8771, 10.6841)
  line L407 (10.8771, 10.6841) -> (13.3706, 7.4123)
  spline S82 degree 2 poles (13.3706, 7.4123) (13.2699, 7.6524) (13.2699, 7.7879) knots 0 0 0 1 1 1
  line L408 (13.2699, 7.7879) -> (13.2699, 10.6841)
  line L409 (13.2699, 10.6841) -> (14.7877, 10.6841)
  line L410 (14.7877, 10.6841) -> (14.7877, 5.4841)
  line L411 (14.7877, 5.4841) -> (13.4248, 5.4841)
  line L412 (13.4248, 5.4841) -> (10.9313, 8.69)
  spline S83 degree 2 poles (10.9313, 8.69) (11.032, 8.45) (11.032, 8.3145) knots 0 0 0 1 1 1
  line L413 (11.032, 8.3145) -> (11.032, 5.4841)
  line L414 (11.032, 5.4841) -> (9.5142, 5.4841)
  line L415 (9.5142, 5.4841) -> (9.5142, 10.6841)
  spline S84 degree 2 poles (3.9192, 10.2698) (3.9192, 10.6841) (4.7633, 10.6841) knots 0 0 0 1 1 1
  line L416 (4.7633, 10.6841) -> (7.4891, 10.6841)
  spline S85 degree 2 poles (7.4891, 10.6841) (8.3448, 10.6841) (8.3448, 10.2698) knots 0 0 0 1 1 1
  line L417 (8.3448, 10.2698) -> (8.3448, 7.7453)
  spline S86 degree 2 poles (8.3448, 7.7453) (8.3448, 7.331) (7.4891, 7.331) knots 0 0 0 1 1 1
  line L418 (7.4891, 7.331) -> (4.7633, 7.331)
  spline S87 degree 2 poles (4.7633, 7.331) (3.9192, 7.331) (3.9192, 7.7453) knots 0 0 0 1 1 1
  line L419 (3.9192, 7.7453) -> (3.9192, 10.2698)
  line L420 (5.406, 10.053) -> (5.406, 7.9621)
  line L421 (5.406, 7.9621) -> (6.8503, 7.9621)
  line L422 (6.8503, 7.9621) -> (6.8503, 10.053)
  line L423 (6.8503, 10.053) -> (5.406, 10.053)
  line L424 (-3.8208, 7.331) -> (-2.3765, 10.6918)
  line L425 (-2.3765, 10.6918) -> (-1.0485, 10.6918)
  line L426 (-1.0485, 10.6918) -> (-0.3244, 8.8333)
  line L427 (-0.3244, 8.8333) -> (0.3996, 10.6918)
  line L428 (0.3996, 10.6918) -> (1.7161, 10.6918)
  line L429 (1.7161, 10.6918) -> (3.1603, 7.331)
  line L430 (3.1603, 7.331) -> (1.7045, 7.331)
  line L431 (1.7045, 7.331) -> (0.9727, 9.4722)
  line L432 (0.9727, 9.4722) -> (0.2486, 7.331)
  line L433 (0.2486, 7.331) -> (-0.9091, 7.331)
  line L434 (-0.9091, 7.331) -> (-1.6331, 9.4722)
  line L435 (-1.6331, 9.4722) -> (-2.3649, 7.331)
  line L436 (-2.3649, 7.331) -> (-3.8208, 7.331)
  line L437 (-8.8969, 10.6841) -> (-7.441, 10.6841)
  line L438 (-7.441, 10.6841) -> (-7.441, 10.5679)
  spline S88 degree 2 poles (-7.441, 10.5679) (-6.926, 10.6066) (-6.4072, 10.6492) knots 0 0 0 1 1 1
  spline S89 degree 2 poles (-6.4072, 10.6492) (-5.7296, 10.6957) (-5.3773, 10.6957) knots 0 0 0 1 1 1
  spline S90 degree 2 poles (-5.3773, 10.6957) (-4.5448, 10.6957) (-4.5448, 10.2891) knots 0 0 0 1 1 1
  line L439 (-4.5448, 10.2891) -> (-4.5448, 9.0811)
  spline S91 degree 2 poles (-4.5448, 9.0811) (-4.5448, 8.6629) (-5.4005, 8.6629) knots 0 0 0 1 1 1
  line L440 (-5.4005, 8.6629) -> (-7.4565, 8.6629)
  line L441 (-7.4565, 8.6629) -> (-7.4565, 7.8924)
  line L442 (-7.4565, 7.8924) -> (-6.0007, 7.8924)
  line L443 (-6.0007, 7.8924) -> (-6.0007, 8.3725)
  line L444 (-6.0007, 8.3725) -> (-4.6261, 8.3725)
  line L445 (-4.6261, 8.3725) -> (-4.6261, 7.7453)
  spline S92 degree 2 poles (-4.6261, 7.7453) (-4.6261, 7.331) (-5.4818, 7.331) knots 0 0 0 1 1 1
  line L446 (-5.4818, 7.331) -> (-8.0528, 7.331)
  spline S93 degree 2 poles (-8.0528, 7.331) (-8.8969, 7.331) (-8.8969, 7.7453) knots 0 0 0 1 1 1
  line L447 (-8.8969, 7.7453) -> (-8.8969, 10.6841)
  line L448 (-7.4565, 10.0801) -> (-7.4565, 9.1779)
  line L449 (-7.4565, 9.1779) -> (-6.0007, 9.1779)
  line L450 (-6.0007, 9.1779) -> (-6.0007, 10.1072)
  line L451 (-6.0007, 10.1072) -> (-7.4565, 10.0801)
  line L452 (-14.2208, 8.7326) -> (-12.7146, 8.7326)
  line L453 (-12.7146, 8.7326) -> (-12.7146, 7.9621)
  line L454 (-12.7146, 7.9621) -> (-11.5104, 7.9776)
  line L455 (-11.5104, 7.9776) -> (-11.5104, 10.6841)
  line L456 (-11.5104, 10.6841) -> (-9.9887, 10.6841)
  line L457 (-9.9887, 10.6841) -> (-9.9887, 7.331)
  line L458 (-9.9887, 7.331) -> (-11.5104, 7.331)
  line L459 (-11.5104, 7.331) -> (-11.5104, 7.451)
  spline S94 degree 2 poles (-11.5104, 7.451) (-11.9828, 7.4084) (-12.4474, 7.3658) knots 0 0 0 1 1 1
  spline S95 degree 2 poles (-12.4474, 7.3658) (-13.0127, 7.3155) (-13.3922, 7.3155) knots 0 0 0 1 1 1
  spline S96 degree 2 poles (-13.3922, 7.3155) (-14.2208, 7.3155) (-14.2208, 7.7259) knots 0 0 0 1 1 1
  line L460 (-14.2208, 7.7259) -> (-14.2208, 8.7326)
  line L461 (-19.5602, 10.6841) -> (-17.9378, 10.6841)
  line L462 (-17.9378, 10.6841) -> (-16.602, 9.1469)
  line L463 (-16.602, 9.1469) -> (-16.602, 10.6841)
  line L464 (-16.602, 10.6841) -> (-15.0803, 10.6841)
  line L465 (-15.0803, 10.6841) -> (-15.0803, 5.4841)
  line L466 (-15.0803, 5.4841) -> (-16.602, 5.4841)
  line L467 (-16.602, 5.4841) -> (-16.602, 8.6087)
  line L468 (-16.602, 8.6087) -> (-17.8062, 7.331)
  line L469 (-17.8062, 7.331) -> (-19.3937, 7.331)
  line L470 (-19.3937, 7.331) -> (-19.3937, 7.3426)
  line L471 (-19.3937, 7.3426) -> (-17.8449, 8.8682)
  line L472 (-17.8449, 8.8682) -> (-19.5602, 10.6841)
  line L473 (-21.7478, 10.6841) -> (-20.2532, 10.6841)
  line L474 (-20.2532, 10.6841) -> (-20.2532, 7.331)
  line L475 (-20.2532, 7.331) -> (-21.7478, 7.331)
  line L476 (-21.7478, 7.331) -> (-21.7478, 10.6841)
  line L477 (-21.7633, 6.847) -> (-20.2416, 6.847)
  line L478 (-20.2416, 6.847) -> (-20.2416, 6.0649)
  line L479 (-20.2416, 6.0649) -> (-21.7633, 6.0649)
  line L480 (-21.7633, 6.0649) -> (-21.7633, 6.847)
  spline S97 degree 2 poles (-27.2227, 10.2698) (-27.2227, 10.6841) (-26.3631, 10.6841) knots 0 0 0 1 1 1
  line L481 (-26.3631, 10.6841) -> (-23.738, 10.6841)
  spline S98 degree 2 poles (-23.738, 10.6841) (-22.8823, 10.6841) (-22.8823, 10.2698) knots 0 0 0 1 1 1
  line L482 (-22.8823, 10.2698) -> (-22.8823, 7.7453)
  spline S99 degree 2 poles (-22.8823, 7.7453) (-22.8823, 7.331) (-23.738, 7.331) knots 0 0 0 1 1 1
  line L483 (-23.738, 7.331) -> (-26.3631, 7.331)
  spline S100 degree 2 poles (-26.3631, 7.331) (-27.2227, 7.331) (-27.2227, 7.7453) knots 0 0 0 1 1 1
  line L484 (-27.2227, 7.7453) -> (-27.2227, 8.9766)
  line L485 (-27.2227, 8.9766) -> (-26.8045, 9.1856)
  line L486 (-26.8045, 9.1856) -> (-24.3381, 9.1856)
  line L487 (-24.3381, 9.1856) -> (-24.3381, 10.1265)
  line L488 (-24.3381, 10.1265) -> (-25.7669, 10.1265)
  line L489 (-25.7669, 10.1265) -> (-25.7669, 9.569)
  line L490 (-25.7669, 9.569) -> (-27.2227, 9.569)
  line L491 (-27.2227, 9.569) -> (-27.2227, 10.2698)
  line L492 (-25.7669, 8.69) -> (-25.7669, 7.8886)
  line L493 (-25.7669, 7.8886) -> (-24.3381, 7.8886)
  line L494 (-24.3381, 7.8886) -> (-24.3381, 8.69)
  line L495 (-24.3381, 8.69) -> (-25.7669, 8.69)
  line L496 (-34.9666, 7.331) -> (-33.5223, 10.6918)
  line L497 (-33.5223, 10.6918) -> (-32.1943, 10.6918)
  line L498 (-32.1943, 10.6918) -> (-31.4702, 8.8333)
  line L499 (-31.4702, 8.8333) -> (-30.7462, 10.6918)
  line L500 (-30.7462, 10.6918) -> (-29.4297, 10.6918)
  line L501 (-29.4297, 10.6918) -> (-27.9855, 7.331)
  line L502 (-27.9855, 7.331) -> (-29.4413, 7.331)
  line L503 (-29.4413, 7.331) -> (-30.1731, 9.4722)
  line L504 (-30.1731, 9.4722) -> (-30.8972, 7.331)
  line L505 (-30.8972, 7.331) -> (-32.0549, 7.331)
  line L506 (-32.0549, 7.331) -> (-32.7789, 9.4722)
  line L507 (-32.7789, 9.4722) -> (-33.5107, 7.331)
  line L508 (-33.5107, 7.331) -> (-34.9666, 7.331)
  line L509 (-37.251, 10.6841) -> (-35.7564, 10.6841)
  line L510 (-35.7564, 10.6841) -> (-35.7564, 7.331)
  line L511 (-35.7564, 7.331) -> (-37.251, 7.331)
  line L512 (-37.251, 7.331) -> (-37.251, 10.6841)
  line L513 (-37.2665, 6.847) -> (-35.7448, 6.847)
  line L514 (-35.7448, 6.847) -> (-35.7448, 6.0649)
  line L515 (-35.7448, 6.0649) -> (-37.2665, 6.0649)
  line L516 (-37.2665, 6.0649) -> (-37.2665, 6.847)
  spline S101 degree 2 poles (-42.7259, 10.2698) (-42.7259, 10.6841) (-41.8818, 10.6841) knots 0 0 0 1 1 1
  line L517 (-41.8818, 10.6841) -> (-39.2412, 10.6841)
  spline S102 degree 2 poles (-39.2412, 10.6841) (-38.3855, 10.6841) (-38.3855, 10.2698) knots 0 0 0 1 1 1
  line L518 (-38.3855, 10.2698) -> (-38.3855, 7.7453)
  spline S103 degree 2 poles (-38.3855, 7.7453) (-38.3855, 7.331) (-39.2412, 7.331) knots 0 0 0 1 1 1
  line L519 (-39.2412, 7.331) -> (-41.8818, 7.331)
  spline S104 degree 2 poles (-41.8818, 7.331) (-42.7259, 7.331) (-42.7259, 7.7453) knots 0 0 0 1 1 1
  line L520 (-42.7259, 7.7453) -> (-42.7259, 8.5429)
  line L521 (-42.7259, 8.5429) -> (-41.243, 8.5429)
  line L522 (-41.243, 8.5429) -> (-41.243, 7.9621)
  line L523 (-41.243, 7.9621) -> (-39.88, 7.9621)
  line L524 (-39.88, 7.9621) -> (-39.88, 10.053)
  line L525 (-39.88, 10.053) -> (-41.243, 10.053)
  line L526 (-41.243, 10.053) -> (-41.243, 9.4102)
  line L527 (-41.243, 9.4102) -> (-42.7259, 9.4102)
  line L528 (-42.7259, 9.4102) -> (-42.7259, 10.2698)
  line L529 (-47.6123, 10.6841) -> (-43.57, 10.6841)
  line L530 (-43.57, 10.6841) -> (-43.57, 10.2349)
  line L531 (-43.57, 10.2349) -> (-45.8041, 7.9505)
  line L532 (-45.8041, 7.9505) -> (-43.752, 7.9505)
  line L533 (-43.752, 7.9505) -> (-43.752, 7.331)
  line L534 (-43.752, 7.331) -> (-47.6123, 7.331)
  line L535 (-47.6123, 7.331) -> (-47.6123, 7.7801)
  line L536 (-47.6123, 7.7801) -> (-45.3666, 10.0646)
  line L537 (-45.3666, 10.0646) -> (-47.6123, 10.0646)
  line L538 (-47.6123, 10.0646) -> (-47.6123, 10.6841)
  point P0 (0, 0)
  constraints: 2 other
extrude "Extrusion2" add sketch "Sketch2" along normal blind 1.2
sketch "Sketch3" plane through (0, 2, 0) normal (0, 1, 0) x (1, 0, 0)
  line L0 (75, -5) -> (75, 15) projected
  line L1 (-75, 15) -> (-75, -5) projected
  circle A0 centre (-60, 0) radius 1.5
  circle A1 centre (60, 0) radius 1.5
  point P0 (0, 0)
  dimension "d9" = 3
  dimension "d10" = 3
  dimension "d11" = 15
  dimension "d12" = 15
  constraints: 2 centre point
  measures "d9" diameter of A0
  measures "d10" diameter of A1
  measures "d11" distance from line of A0.centre L1
  measures "d12" distance from line of L0 A1.centre
extrude "Extrusion3" cut sketch "Sketch3" against normal blind 1.2
body "Solid1"
